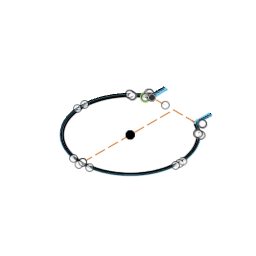
E-Baike Kunstoff abdeckung Schloss v11 (Autodesk Fusion 360 design; units mm, degrees)
Autodesk Fusion 360 part; units mm, degrees
sketch "Skizze3" plane through (0, 0, 0) normal (0, 0, 1) x (1, 0, 0)
  line L0 (52.5263, 0.0019) -> (52.3815, 0.0019) construction
  line L1 (52.3815, 0.0019) -> (52.3815, -3.9178)
  line L2 (52.3815, 0.0019) -> (52.3815, 3.8983)
  line L3 (0, -50.55) -> (0, -54.6366)
  arc A0 (37.2241, 37.4698) -> (37.51, 36.7698) centre (38.2241, 37.4698) ccw
  arc A1 (34.4473, 37.4285) -> (34.7597, 36.7024) centre (35.4473, 37.4285) ccw
  line L4 (-52.3815, 0.0019) -> (-52.3815, -3.9178)
  line L5 (-52.3815, 0.0019) -> (-52.3815, 3.8983)
  arc A2 (-34.7597, 36.7024) -> (-34.4473, 37.4285) centre (-35.4473, 37.4285) ccw
  arc A3 (-37.51, 36.7698) -> (-37.2241, 37.4698) centre (-38.2241, 37.4698) ccw
  line L6 (0, -50.55) -> (0, 46.165) construction
  line L7 (-25.0003, 48.4886) -> (-24.9973, 61.165)
  line L8 (25.0009, 48.4892) -> (25.0009, 61.165)
  line L9 (-24.9973, 61.165) -> (-24.3973, 61.1649)
  line L10 (25.0009, 61.165) -> (24.4009, 61.165)
  line L11 (23.8294, 48.6654) -> (24.4009, 61.165)
  line L12 (-23.8287, 48.6648) -> (-24.3973, 61.1649)
  line L13 (24.4009, 61.165) -> (22.5009, 61.165)
  line L14 (-24.3973, 61.1649) -> (-22.4973, 61.1644)
  arc A4 (-26.748, 42.8934) -> (-26.748, 42.8934) centre (0, 0) ccw
  arc A5 (-25.8336, 45.0137) -> (25.8341, 45.0134) centre (0, 0) ccw
  line L15 (-8.6883, 46.1611) -> (-20.5959, 46.164) construction
  line L16 (0, 46.165) -> (20.5936, 46.165) construction
  arc A6 (-25.8336, 45.0137) -> (-23.8287, 48.6648) centre (-27.8246, 48.483) ccw
  arc A7 (-26.9472, 45.0566) -> (-25.0003, 48.4886) centre (-29.0003, 48.4895) ccw
  arc A8 (25.0009, 48.4892) -> (26.9477, 45.0563) centre (29.0009, 48.4892) ccw
  arc A9 (23.8294, 48.6654) -> (25.8341, 45.0134) centre (27.8252, 48.4827) ccw
  line L17 (20.5936, 46.165) -> (22.0936, 46.165) construction
  line L18 (-20.5959, 46.164) -> (-22.0959, 46.164) construction
  line L19 (22.0936, 46.165) -> (22.0936, 45.4662) construction
  line L20 (-22.0959, 46.164) -> (-22.0959, 45.4651) construction
  line L21 (22.1899, 49.1795) -> (22.5009, 61.165)
  line L22 (-22.1908, 49.1767) -> (-22.4973, 61.1644)
  arc A10 (-25.198, 43.822) -> (25.1971, 43.8224) centre (0, 0) ccw
  arc A11 (52.3815, 3.5258) -> (26.9477, 45.0563) centre (0, 0) ccw
  arc A12 (-26.9472, 45.0566) -> (-52.3815, 3.5258) centre (0, 0) ccw
  arc A13 (-52.3815, -3.5258) -> (52.3815, -3.5258) centre (0, 0) ccw
  arc A14 (-25.198, 43.822) -> (-22.1908, 49.1767) centre (-28.1889, 49.0234) ccw
  arc A15 (22.1899, 49.1795) -> (25.1971, 43.8224) centre (28.1879, 49.0239) ccw
  line L23 (8.6033, -51.817) -> (8.6033, -51.7903) construction
  line L24 (-8.6033, -51.817) -> (-8.6033, -51.7903) construction
  point P0 (-25.0009, 46.165)
  point P1 (-25.0009, 46.165)
  point P2 (-25.7438, 46.1667)
  point P3 (-22.9574, 46.0854)
  dimension "d26" = 1
  dimension "d34" = 105
  dimension "d36" = 96.715
  dimension "d42" = 15
  dimension "d44" = 2.5
  dimension "d45" = 2.5
  dimension "d46" = 0.6
  dimension "d47" = 0.6
  dimension "d48" = 103.8
  dimension "d50" = 4
  dimension "d57" = 101.1
  dimension "d58" = 1.5
  dimension "d59" = 1.5
  dimension "d61" = 6
  dimension "d62" = 6
  constraint horizontal L0
  constraint perpendicular L0 L1
  constraint perpendicular L0 L2
  constraint vertical L3
  constraint equal A0 A1
  constraint symmetric L0.end L3 L4.start
  constraint symmetric L1.end L3 L4.end
  constraint symmetric L2.end L3 L5.end
  constraint symmetric L3 A0.start A3.end
  constraint symmetric L3 A0.end A3.start
  constraint symmetric L3 A0 A3
  constraint symmetric L3 A1.start A2.end
  constraint symmetric L3 A1.end A2.start
  constraint symmetric L3 A1 A2
  constraint symmetric L3 L23.start L24.start
  constraint parallel L3 L6
  constraint coincident A4.centre A5.centre
  constraint perpendicular L6 L16
  constraint perpendicular L7 L15
  constraint perpendicular L8 L16
  constraint perpendicular L7 L9
  constraint perpendicular L8 L10
  constraint parallel L10 L13
  constraint parallel L9 L14
  constraint coincident A4 L15.end
  constraint tangent A5 A6
  constraint tangent L12 A6
  constraint tangent A7 A12
  constraint tangent L7 A7
  constraint equal A6 A7
  constraint tangent A8 A12
  constraint tangent L8 A8
  constraint equal A6 A8
  constraint tangent A5 A9
  constraint tangent L11 A9
  constraint equal A6 A9
  constraint coincident A7 P2
  constraint concentric A5 A10
  constraint parallel L16 L17
  constraint perpendicular L6 L18
  constraint perpendicular L17 L19
  constraint perpendicular L18 L20
  constraint coincident L20.end L22
  constraint coincident L20.end A10
  constraint coincident L19.end L21
  constraint coincident L19.end A10
  constraint coincident L1 A13.end
  constraint concentric A11 A12
  constraint coincident L2 A11.start
  constraint coincident L5 A12.end
  constraint coincident L4 A13.start
  constraint concentric A12 A13
  constraint tangent A10 A14
  constraint tangent L22 A14
  constraint midpoint A14 P3
  constraint tangent A10 A15
  constraint tangent L21 A15
  constraint coincident A13 L23.end
  constraint vertical L23
  constraint coincident A13 L24.end
  constraint vertical L24
  measures "d26" radius of A0
  measures "d34" diameter of A12
  measures "d36" distance of L3.start L6.end
  measures "d42" distance of P1 L7.end
  measures "d44" distance of L8.end L13.end
  measures "d45" distance of L7.end L14.end
  measures "d46" distance of L7.end L9.end
  measures "d47" distance of L8.end L10.end
  measures "d48" diameter of A5
  measures "d50" radius of A6
  measures "d57" diameter of A10
  measures "d58" distance of L16.end L17.end
  measures "d59" distance of L15.end L18.end
  measures "d61" radius of A14
  measures "d62" radius of A15
sketch "Skizze6" plane through (0, 0, 0) normal (0, 0, 1) x (1, 0, 0)
sketch "Skizze7" plane through (0, 0, 0) normal (0, 0, 1) x (1, 0, 0)
sketch "Skizze8" plane through (0, 0, 0) normal (0, 0, 1) x (1, 0, 0)
sketch "Skizze9" plane through (0, 0, 0) normal (0, 0, 1) x (1, 0, 0)
sketch "Skizze5" plane through (0, 0, 0) normal (0, 0, 1) x (1, 0, 0)
extrude "Extrusion4" add sketch "Skizze3" along normal blind 1.2 contours L1 L2 L3 L8 L10 L11 A5 A8 A9 A11 A13 | L3 L4 L5 L7 L9 L12 A5 A6 A7 A12 A13
ref_plane "Arbeitsebene1" through (-30.2101, 4.6324, 1) normal (0, 0, 1) x (1, 0, 0)
ref_plane "Arbeitsebene2" through (30.2101, 4.6325, 1) normal (0, 0, 1) x (1, 0, 0)
sketch "Skizze10" plane through (0, 0, 1) normal (0, 0, 1) x (1, 0, 0)
sketch "Skizze4" plane through (0, 0, 0) normal (0, 0, 1) x (1, 0, 0)
